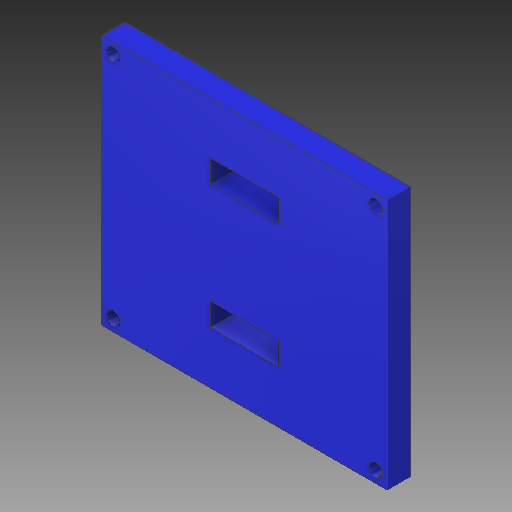
# Autodesk Inventor part: support_card
Saved by Autodesk Inventor 2019 (Build 230136000, 136)
## iProperties
Created: 2018-09-21
Part Number: support_card
Material: Générique
Document SubType Name: Modeling
Designer: Jérémy
Density: 1 g/cm^3
Appearance: Par défaut
Author: Jérémy
Autodesk Inventor part; units mm, degrees
ref_plane "YZ Plane" through (0, 0, 0) normal (1, 0, 0) x (0, 1, 0)
ref_plane "XZ Plane" through (0, 0, 0) normal (0, 1, 0) x (-1, 0, 0)
ref_plane "XY Plane" through (0, 0, 0) normal (0, 0, 1) x (1, 0, 0)
sketch "Esquisse1" plane through (0, 0, 0) normal (0, 0, 1) x (1, 0, 0)
  circle A0 centre (28.6, 24.9) radius 1.5 projected
  circle A1 centre (28.6, -24.9) radius 1.5 projected
  circle A2 centre (-28.6, 24.9) radius 1.5 projected
  circle A3 centre (-28.6, -24.9) radius 1.5 projected
  line L0 (31.1, 27.4) -> (-31.1, 27.4) projected
  line L1 (-31.1, 27.4) -> (-31.1, -27.4) projected
  line L2 (-31.1, -27.4) -> (31.1, -27.4) projected
  line L3 (31.1, -27.4) -> (31.1, 27.4) projected
  line L4 (-7.5, 16) -> (0, 16)
  line L5 (0, 16) -> (7.5, 16)
  line L6 (7.5, 16) -> (7.5, 11)
  line L7 (7.5, 11) -> (0, 11)
  line L8 (0, 11) -> (-7.5, 11)
  line L9 (-7.5, 11) -> (-7.5, 16)
  line L10 (0, 37.051) -> (0, -38.1524) construction
  line L11 (34.7968, 0) -> (-21.7073, 0) construction
  line L12 (-7.5, -16) -> (0, -16)
  line L13 (0, -16) -> (7.5, -16)
  line L14 (7.5, -16) -> (7.5, -11)
  line L15 (7.5, -11) -> (0, -11)
  line L16 (0, -11) -> (-7.5, -11)
  line L17 (-7.5, -11) -> (-7.5, -16)
  line L18 (0, -37.051) -> (0, 38.1524) construction
  point P0 (0, 0)
  point P1 (0, 27.4)
  point P2 (31.1, 0)
  dimension "d0" = 7.5
  dimension "d1" = 16
  dimension "d2" = 5
  constraints: 30 end point, 8 point on line, 8 symmetric about line, 3 perpendicular, 2 collinear, 2 horizontal, 2 midpoint, 1 vertical
  measures "d0" distance of L4.end L5.end
  measures "d1" vertical distance of L5.end point (0, 0)
  measures "d2" distance of L5.end L6.end
extrude "Extrusion1" add sketch "Esquisse1" along normal blind 5
equation "\"d0\" = 0.5 * L_attache_carte"
equation "\"d1\" = 0.5 * largeur"
equation "\"d2\" = epaisseur"
equation "\"d3\" = epaisseur"
equation "\"epaisseur\" = 5"
equation "\"dvis\" = 3"
equation "\"largeur\" = 32"
equation "\"L_attache_carte\" = 15"
equation "\"marge_attache_carte\" = 5"
equation "\"L_cubi\" = 76.6"
equation "\"taille_trou\" = 7"
equation "\"L_moteur\" = 28.3"
equation "\"marge_trou\" = 2"
equation "\"largeur_cubi\" = 76.6"
